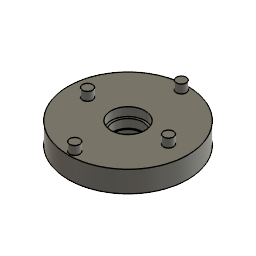
magnet zigu (Autodesk Fusion 360 design; units mm, degrees)
Autodesk Fusion 360 part; units mm, degrees
sketch "スケッチ1" plane through (0, 0, 0) normal (0, 1, 0) x (1, 0, 0)
  circle A0 centre (0, 0) radius 14
  circle A1 centre (0, 0) radius 9.5 construction
  line L0 (-9.5, 0) -> (9.5, 0) construction
  circle A2 centre (-9.5, 0) radius 1.175
  circle A3 centre (9.5, 0) radius 1.175
  circle A4 centre (0, 0) radius 12.5 construction
  line L1 (0, 12.5) -> (0, -12.5) construction
  circle A5 centre (0, 12.5) radius 1.175
  circle A6 centre (0, -12.5) radius 1.175
  dimension "d1" = 28
  dimension "d2" = 19
  dimension "d3" = 2.35
  dimension "d4" = 2.35
  dimension "d5" = 25
  dimension "d6" = 2.35
  dimension "d7" = 2.35
  constraint coincident A0.centre A1.centre
  constraint coincident A1 L0.start
  constraint coincident A1 L0.end
  constraint horizontal L0
  constraint coincident A0.centre L0
  constraint coincident L0.start A2.centre
  constraint coincident L0.end A3.centre
  constraint concentric A0 A4
  constraint coincident A4 L1.start
  constraint coincident A4 L1.end
  constraint vertical L1
  constraint coincident A0.centre L1
  constraint coincident L1.start A5.centre
  constraint coincident L1.end A6.centre
  measures "d1" diameter of A0
  measures "d2" diameter of A1
  measures "d3" diameter of A2
  measures "d4" diameter of A3
  measures "d5" diameter of A4
  measures "d6" diameter of A5
  measures "d7" diameter of A6
extrude "押し出し1" add sketch "スケッチ1" along normal blind 2 contours A2 | A3 | A5 | A6 makes body 1 at (-8.3265, 1.3333, 0.0586) makes body 2 at (10.6735, 1.3333, 0.0586) makes body 3 at (1.1735, 1.3333, -12.4414) makes body 4 at (1.1735, 1.3333, 12.5586)
extrude "押し出し2" add sketch "スケッチ1" against normal blind 4 contours A0 | A2 | A3 | A5 | A6 bodies 1 2 3 4
sketch "スケッチ2" plane through (0, -4, 0) normal (0, -1, 0) x (1, 0, 0)
  circle A0 centre (0, 0) radius 14
  circle A1 centre (0, 0) radius 4
  dimension "d12" = 8
  constraint coincident A0.centre A1.centre
  measures "d12" diameter of A1
extrude "押し出し3" cut sketch "スケッチ2" against normal blind 4 contours A1 bodies 1
ref_plane "作業平面1" through (0, -2, 0) normal (0, -1, 0) x (-1, 0, 0)
sketch "スケッチ3" plane through (0, -2, 0) normal (0, -1, 0) x (-1, 0, 0)
  circle A0 centre (0, 0) radius 4
  circle A1 centre (0, 0) radius 3.45
  dimension "d16" = 8
  dimension "d17" = 6.9
  constraint coincident A0.centre A1.centre
  constraint concentric A0 A1
  measures "d16" diameter of A0
  measures "d17" diameter of A1
extrude "押し出し4" add sketch "スケッチ3" along normal blind 3 bodies 1
ref_plane "作業平面3" through (0, -4, 0) normal (0, -1, 0) x (-1, 0, 0)
sketch "スケッチ5" plane through (0, -4, 0) normal (0, -1, 0) x (-1, 0, 0)
  circle A0 centre (0, 0) radius 3.45
  circle A1 centre (0, 0) radius 3.15
  dimension "d26" = 6.9
  dimension "d27" = 6.3
  constraint coincident A0.centre A1.centre
  measures "d26" diameter of A0
  measures "d27" diameter of A1
extrude "押し出し6" add sketch "スケッチ5" along normal blind 1 bodies 1
extrude "押し出し7" add 1 faces at (10.6145, -4, 0.6955) along direction (0, -1, 0) blind 1 on bodies 1 bodies 1
